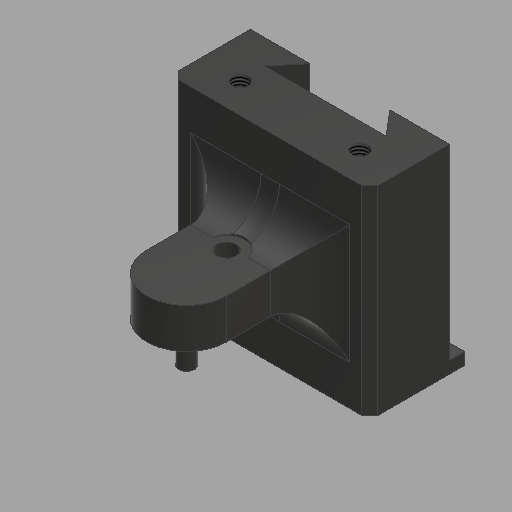
# Autodesk Inventor part: BT401_trajan20_21
Saved by Autodesk Inventor 2023 (Build 270158000, 158)
## iProperties
Company: HTBLA Kaindorf
RuleStatus: InUse
Created: 2022-08-07
Part Number: BT401_trajan20_21
Project: Zeichenmaschine_v2
Material: Kunststoff, undurchsichtig Schwarz
Description: Stifthalter außen
Document SubType Name: Modeling
Designer: trajan20
Density: 0.952 g/cm^3
Appearance: Glatt - Schwarz
Mass: 47.3739 g
Surface Area: 127.143 cm^2
Volume: 49.7625 cm^3
AfterDocNew0: iProperties-Editor_aufrufen
Haupt_Länge: 50,000 mm
Einkerbung_Breite: 30,000 mm
Einkerbung_Winkel_Außen: 50,00 grd
Einkerbung_Tiefe: 6,000 mm
Haupt_Breite: 20,000 mm
Federn_Abstand_Breite: 10,000 mm
Federn_Abstand_Länge: 7,500 mm
Haupt_Höhe: 50,000 mm
Author: jan
Keywords: 2021
Autodesk Inventor part; units mm, degrees
ref_plane "YZ Plane" through (0, 0, 0) normal (1, 0, 0) x (0, 1, 0)
ref_plane "XZ Plane" through (0, 0, 0) normal (0, 1, 0) x (-1, 0, 0)
ref_plane "XY Plane" through (0, 0, 0) normal (0, 0, 1) x (1, 0, 0)
sketch "Skizze3" plane through (0, 0, 0) normal (0, 0, 1) x (1, 0, 0)
  circle A0 centre (0, 0) radius 2.5
  circle A1 centre (10, 0) radius 2
  line L0 (0, -35) -> (0, 35) projected
  line L1 (-41.2, 0) -> (30.2, 0) projected
  arc A2 (10, -10) -> (10, 10) centre (10, 0) ccw
  line L2 (10, -10) -> (0, -10)
  line L3 (10, 10) -> (0, 10)
  arc A3 (0, 10) -> (0, -10) centre (0, 0) ccw
  line L4 (0, -10) -> (-11, -10)
  line L5 (0, 10) -> (-11, 10)
  line L6 (-11, -10) -> (-11, -25)
  line L7 (-11, -25) -> (-31, -25)
  line L8 (-31, -25) -> (-31, 25)
  line L9 (-31, 25) -> (-11, 25)
  line L10 (-11, 25) -> (-11, 10)
  line L11 (-31, -10.0476) -> (-24.8, -15.25)
  line L12 (-24.8, -15.25) -> (-24.8, 15.25)
  line L13 (-24.8, 15.25) -> (-31, 10.0476)
  line L14 (-11, -10) -> (-11, 10)
  point P0 (-10, 0)
  point P1 (-31, 0)
  dimension "d5" = 5
  dimension "d6" = 4
  dimension "d7" = 10
  dimension "d8" = 20
  dimension "d10" = 10
  dimension "d11" = 50
  dimension "d13" = 11
  dimension "d17" = 6.2
  dimension "d19" = 30.5
  dimension "d43" = 20
  dimension "d44" = 50
  dimension "d54" = 20.0952
  constraints: 26 end point, 7 point on line, 5 perpendicular, 4 centre point, 4 point on circle, 3 coincident, 3 tangent, 2 horizontal, 1 midpoint, 1 parallel, 1 vertical, 1 other
  measures "d5" diameter of A0
  measures "d6" diameter of A1
  measures "d7" distance from line of L0 A1.centre
  measures "d8" diameter of A2
  measures "d10" radius of A3
  measures "d11" angle of L8 L11
  measures "d13" distance of L2.end L4.end
  measures "d17" distance between parallel lines of L8 L12
  measures "d19" distance of L11.end L12.end
  measures "d43" distance between parallel lines of L8 L6
  measures "d44" distance between parallel lines of L9 L7
  measures "d54" distance of L13.end L11.start
extrude "Extrusion3" add sketch "Skizze3" along normal mid plane 10 contours L1 A1 A2 L2 L0 A0 | A0 L0 L3 A2 L1 A1 | A0 L1 A3 L0 | L0 A3 L1 A0 | L1 A1 | A1 L1 | A3 L1 L14 L5 | L4 L14 L1 A3
extrude "Extrusion4" add sketch "Skizze3" along normal mid plane 50 contours L14 L1 L12 L13 L8 L9 L10 | L6 L7 L8 L11 L12 L1 L14
chamfer "Fase1" distance 2 angle 45 2 edges at (-11, 25, 0) (-11, -25, 0)
fillet "Rundung1" radius 10 4 edges at (-11, 0, 5) (-11, -10, 0) (-11, 0, -5) (-11, 10, 0)
sketch "Skizze5" plane through (0, 0, 25) normal (0, 0, 1) x (1, 0, 0)
  line L0 (-31, -25) -> (-13, -25) projected
  line L1 (-11, -23) -> (-11, 23) projected
  line L2 (-13, 25) -> (-31, 25) projected
  point P0 (0, 0)
  point P1 (-18.5, 15)
  point P2 (-18.5, -15)
  dimension "d30" = 10
  dimension "d31" = 7.5
  dimension "d32" = 10
  dimension "d33" = 7.5
  measures "d30" distance from line of L0 point (-18.5, -15)
  measures "d31" distance from line of L1 point (-18.5, -15)
  measures "d32" distance from line of L2 point (-18.5, 15)
  measures "d33" distance from line of L1 point (-18.5, 15)
hole "Bohrung1" at (-18.5, 15, 25) at (-18.5, -15, 25) direction (0, 0, -1) diameter 4.134 depth 15 thread size "M5x0.8" class "6H" standard "ISO Metric profile"
sketch "Skizze6" plane through (0, 0, -5) normal (0, 0, -1) x (-1, 0, 0)
  line L0 (-10, -10) -> (1, -10) projected
  circle A0 centre (0, 0) radius 10.5
  dimension "d47" = 21
  constraints: 1 centre point, 1 coincident
  measures "d47" diameter of A0
extrude "Extrusion6" cut sketch "Skizze6" along normal blind 10
sketch "Skizze7" plane through (0, 0, 5) normal (0, 0, 1) x (1, 0, 0)
  circle A0 centre (0, 0) radius 4.5
  dimension "d48" = 9
  constraints: 1 centre point, 1 coincident
  measures "d48" diameter of A0
extrude "Extrusion7" cut sketch "Skizze7" along normal blind 10
extrude "Extrusion5" add sketch "Skizze3" against normal blind 15 contours L1 A1 | A1 L1
sketch "Skizze8" plane through (-24.8, -15.25, 25) normal (-1, 0, 0) x (0, 0, 1)
  line L0 (-50, -9.75) -> (0, -9.75) projected
  line L1 (-50, 40.25) -> (0, 40.25) projected
  line L2 (-50, -9.75) -> (-47, -9.75)
  line L3 (-47, -9.75) -> (-47, 40.25)
  line L4 (-47, 40.25) -> (-50, 40.25)
  line L5 (-50, 40.25) -> (-50, -9.75)
  point P0 (-25, 15.25)
  dimension "d51" = 3
  constraints: 8 end point, 2 parallel, 1 horizontal, 1 perpendicular, 1 point on line
  measures "d51" distance between parallel lines of L5 L3
extrude "Extrusion8" add sketch "Skizze8" along normal blind 10
equation "\"d11\" = Einkerbung_Winkel_Außen"
equation "\"d43\" = Haupt_Breite"
equation "\"d44\" = Haupt_Länge"
equation "\"d22\" = Haupt_Höhe"
equation "\"d30\" = Federn_Abstand_Breite"
equation "\"d31\" = Federn_Abstand_Länge"
equation "\"d32\" = Federn_Abstand_Breite"
equation "\"d33\" = Federn_Abstand_Länge"
equation "\"Haupt_Länge\" = 50"
equation "\"Einkerbung_Breite\" = 30"
equation "\"Einkerbung_Winkel_Außen\" = 50deg"
equation "\"Einkerbung_Tiefe\" = 6"
equation "\"Haupt_Breite\" = 20"
equation "\"Federn_Abstand_Breite\" = 10"
equation "\"Federn_Abstand_Länge\" = 7.5"
equation "\"Haupt_Höhe\" = 50"
